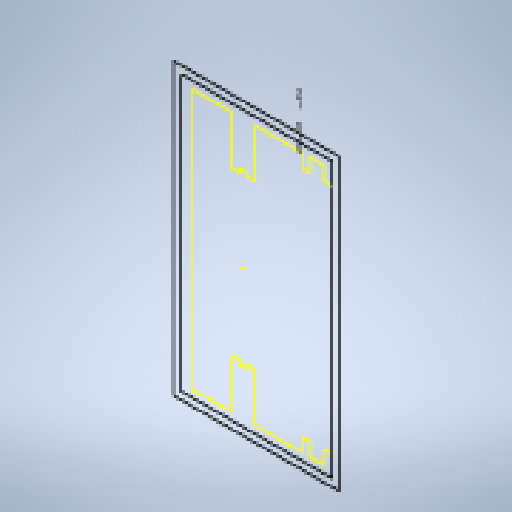
# Autodesk Inventor part: Cache_remote
Saved by Autodesk Inventor 2023 (Build 270158000, 158)
## iProperties
Created: 2023-03-27
Part Number: Cache_remote
Material: Générique
Document SubType Name: Modeling
Designer: eleves
Density: 1 g/cm^3
Appearance: Par défaut
Author: eleves
Autodesk Inventor part; units mm, degrees
ref_plane "YZ Plane" through (0, 0, 0) normal (1, 0, 0) x (0, 1, 0)
ref_plane "XZ Plane" through (0, 0, 0) normal (0, 1, 0) x (-1, 0, 0)
ref_plane "XY Plane" through (0, 0, 0) normal (0, 0, 1) x (1, 0, 0)
sketch "Esquisse1" plane through (0, 0, 0) normal (0, 0, 1) x (1, 0, 0)
  line L0 (-1, -22.45) -> (1, -22.45) projected
  line L1 (-1, -21.45) -> (-1, -22.45) projected
  line L2 (-3, -21.45) -> (-1, -21.45) projected
  line L3 (-3, -21.45) -> (-3, -34.3) projected
  line L4 (-3, -34.3) -> (-13.5643, -34.3) projected
  line L5 (-13.5643, -34.3) -> (-13.5643, 34.3) projected
  line L6 (-13.5643, 34.3) -> (-3, 34.3) projected
  line L7 (-3, 21.45) -> (-3, 34.3) projected
  line L8 (-1, 21.45) -> (-3, 21.45) projected
  line L9 (-1, 22.45) -> (-1, 21.45) projected
  line L10 (1, 22.45) -> (-1, 22.45) projected
  line L11 (1, 21.45) -> (1, 22.45) projected
  line L12 (3, 21.45) -> (1, 21.45) projected
  line L13 (3, 24.45) -> (3, 21.45) projected
  line L14 (3, 24.45) -> (3.0074, 24.45) projected
  line L15 (3.0074, 24.45) -> (3.0074, 34.3) projected
  line L16 (3.0074, 34.3) -> (15.5357, 34.3) projected
  line L17 (15.5357, 34.3) -> (15.5357, 30.7219) projected
  line L18 (15.5357, 30.7219) -> (17.5357, 30.7219) projected
  line L19 (17.5357, 30.7219) -> (17.5357, 34.3) projected
  line L20 (17.5357, 34.3) -> (21.4357, 34.3) projected
  line L21 (21.4357, 34.3) -> (21.4357, 30.7219) projected
  line L22 (21.4357, 30.7219) -> (23.4357, 30.7219) projected
  line L23 (23.4357, 30.7219) -> (23.4357, 36.3) projected
  line L24 (-16.5643, 36.3) -> (23.4357, 36.3) projected
  line L25 (-16.5643, 36.3) -> (-16.5643, -36.3) projected
  line L26 (-16.5643, -36.3) -> (23.4357, -36.3) projected
  line L27 (23.4357, -30.7219) -> (23.4357, -36.3) projected
  line L28 (23.4357, -30.7219) -> (21.4357, -30.7219) projected
  line L29 (21.4357, -30.7219) -> (21.4357, -34.3) projected
  line L30 (21.4357, -34.3) -> (17.5357, -34.3) projected
  line L31 (17.5357, -34.3) -> (17.5357, -30.7219) projected
  line L32 (17.5357, -30.7219) -> (15.5357, -30.7219) projected
  line L33 (15.5357, -30.7219) -> (15.5357, -34.3) projected
  line L34 (15.5357, -34.3) -> (3.0074, -34.3) projected
  line L35 (3.0074, -34.3) -> (3.0074, -24.45) projected
  line L36 (3.0074, -24.45) -> (3, -24.45) projected
  line L37 (3, -21.45) -> (3, -24.45) projected
  line L38 (1, -21.45) -> (3, -21.45) projected
  line L39 (1, -22.45) -> (1, -21.45) projected
  line L40 (23.4357, 36.3) -> (-16.5643, 36.3)
  line L41 (-16.5643, 36.3) -> (-16.5643, -36.3)
  line L42 (-16.5643, -36.3) -> (23.4357, -36.3)
  line L43 (23.4357, -36.3) -> (23.4357, 36.3)
  line L44 (-18.5643, 38.3) -> (25.4357, 38.3)
  line L45 (25.4357, 38.3) -> (25.4357, -38.3)
  line L46 (25.4357, -38.3) -> (-18.5643, -38.3)
  line L47 (-18.5643, -38.3) -> (-18.5643, 38.3)
  point P0 (0, 0)
  dimension "d0" = 2
  constraints: 16 end point, 4 parallel, 2 perpendicular, 1 horizontal, 3 other
  measures "d0" distance between parallel lines of L24 L44
extrude "Extrusion1" add sketch "Esquisse1" along normal blind 2 contours L1 L2 L3 L4 L5 L6 L7 L8 L9 L10 L11 L12 L13 L14 L15 L16 L17 L18 L19 L20 L21 L22 L43 L28 L29 L30 L31 L32 L33 L34 L35 L36 L37 L38 L39 L0 | L0 L39 L38 L37 L36 L35 L34 L33 L32 L31 L30 L29 L28 L27 L26 L25 L24 L23 L22 L21 L20 L19 L18 L17 L16 L15 L14 L13 L12 L11 L10 L9 L8 L7 L6 L5 L4 L3 L2 L1 | L44 L45 L46 L47
sketch "Esquisse2" plane through (0, 0, 0) normal (0, 0, -1) x (-1, 0, 0)
  line L0 (-23.4357, -36.3) -> (-23.4357, 36.3) projected
  line L1 (16.5643, 36.3) -> (-23.4357, 36.3) projected
  line L2 (16.5643, 36.3) -> (16.5643, -36.3) projected
  line L3 (16.5643, -36.3) -> (-23.4357, -36.3) projected
  line L4 (18.5643, -38.3) -> (-25.4357, -38.3) projected
  line L5 (18.5643, 38.3) -> (18.5643, -38.3) projected
  line L6 (-25.4357, 38.3) -> (18.5643, 38.3) projected
  line L7 (-25.4357, -38.3) -> (-25.4357, 38.3) projected
  point P0 (0, 0)
extrude "Extrusion2" add sketch "Esquisse2" along normal blind 2
sketch "Esquisse3" plane through (0, 0, -2) normal (0, 0, -1) x (-1, 0, 0)
  line L0 (-23.4357, -36.3) -> (16.5643, -36.3) construction
  line L1 (16.5643, 36.3) -> (-23.4357, 36.3) construction
  line L2 (16.5643, -36.3) -> (-23.4357, 36.3) construction
  line L3 (-23.4357, -36.3) -> (16.5643, 36.3) construction
  line L4 (-23.9357, 36.7319) -> (17.0643, 36.7319)
  line L5 (17.0643, 36.7319) -> (17.0643, -36.7319)
  line L6 (17.0643, -36.7319) -> (-23.9357, -36.7319)
  line L7 (-23.9357, -36.7319) -> (-23.9357, 36.7319)
  line L8 (-23.9357, 36.7319) -> (17.0643, -36.7319) construction
  line L9 (17.0643, 36.7319) -> (-23.9357, -36.7319) construction
  line L10 (16.5643, 36.3) -> (16.5643, -36.3) projected
  point P0 (0, 0)
  point P1 (-3.4357, 0)
  dimension "d5" = 0.5
  constraints: 16 end point, 3 midpoint, 2 parallel, 1 horizontal, 1 perpendicular
  measures "d5" distance between parallel lines of L10 L5
extrude "Extrusion3" cut sketch "Esquisse3" against normal blind 2
